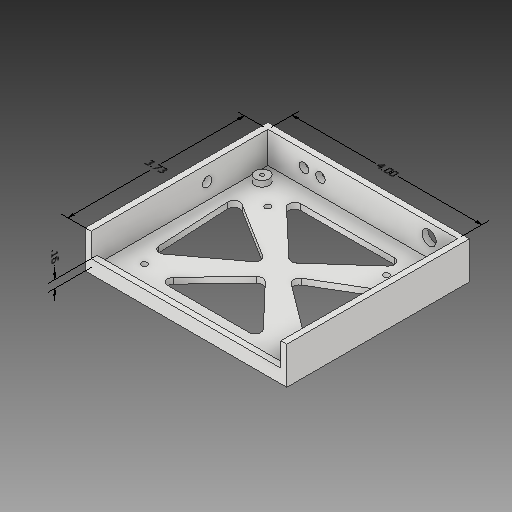
# Autodesk Inventor part: radiocase
Saved by Autodesk Inventor 2018 (Build 220112000, 112)
## iProperties
Created: 2018-03-21
Part Number: radiocase
Material: ABS Plastic
Document SubType Name: Modeling
Designer: Cole Tucker
Density: 1.06 g/cm^3
Appearance: Smooth - White
Mass: 40.9527 g
Surface Area: 278.233 cm^2
Volume: 38.6346 cm^3
Author: Cole Tucker
Autodesk Inventor part; units mm, degrees
ref_plane "YZ Plane" through (0, 0, 0) normal (1, 0, 0) x (0, 1, 0)
ref_plane "XZ Plane" through (0, 0, 0) normal (0, 1, 0) x (-1, 0, 0)
ref_plane "XY Plane" through (0, 0, 0) normal (0, 0, 1) x (1, 0, 0)
sketch "Sketch1" plane through (0, 0, 0) normal (0, 1, 0) x (-1, 0, 0)
  line L0 (0, 0) -> (3.175, 0)
  line L1 (3.175, 0) -> (3.175, -3.175)
  line L2 (3.175, -3.175) -> (0, -3.175)
  line L3 (0, -3.175) -> (0, 0)
  line L4 (3.175, -3.175) -> (104.775, -3.175)
  line L5 (104.775, -3.175) -> (104.775, -94.615)
  line L6 (104.775, -94.615) -> (3.175, -94.615)
  line L7 (3.175, -94.615) -> (3.175, -3.175)
  line L8 (104.775, -94.615) -> (107.95, -94.615)
  line L9 (107.95, -94.615) -> (107.95, -97.79)
  line L10 (107.95, -97.79) -> (104.775, -97.79)
  line L11 (104.775, -97.79) -> (104.775, -94.615)
  line L12 (107.95, -97.79) -> (0, -97.79)
  line L13 (0, -97.79) -> (0, 0)
  line L14 (0, 0) -> (107.95, 0)
  line L15 (107.95, 0) -> (107.95, -97.79)
  dimension "d0" = 3.175
  dimension "d1" = 3.175
  dimension "d2" = 101.6
  dimension "d3" = 91.44
  dimension "d4" = 3.175
  dimension "d5" = 3.175
  constraints: 32 end point, 8 parallel, 4 horizontal, 4 perpendicular
  measures "d0" distance of L1.end L2.end
  measures "d1" distance of L0.end L1.end
  measures "d2" distance of L5.end L6.end
  measures "d3" distance of L4.end L5.end
  measures "d4" distance of L9.end L10.end
  measures "d5" distance of L8.end L9.end
extrude "Extrusion1" add sketch "Sketch1" along normal blind 20 contours L0 L1 L2 L3 | L14 L15 L8 L5 L4 L1 | L2 L7 L6 L11 L12 L13 | L9 L10 L11 L8
sketch "Sketch6" plane through (0, 0, 0) normal (0, -1, 0) x (1, 0, 0)
  line L0 (-104.775, -3.175) -> (-3.175, -3.175) projected
  line L1 (-3.175, -3.175) -> (-3.175, -94.615) projected
  line L2 (-3.175, -94.615) -> (-104.775, -94.615) projected
  line L3 (-104.775, -94.615) -> (-104.775, -3.175) projected
  line L4 (0, 0) -> (0, -97.79) projected
  line L5 (-107.95, 0) -> (0, 0) projected
  line L6 (-107.95, -97.79) -> (-107.95, 0) projected
  line L7 (0, -97.79) -> (-107.95, -97.79) projected
extrude "Extrusion5" add sketch "Sketch6" against normal blind 3.175 contours L0 L1 L2 L3
sketch "Sketch7" plane through (0, 20, 0) normal (0, 1, 0) x (1, 0, 0)
  line L0 (-104.775, 3.175) -> (-3.175, 3.175)
  line L1 (-3.175, 3.175) -> (-3.175, 0)
  line L2 (-3.175, 0) -> (-104.775, 0)
  line L3 (-104.775, 0) -> (-104.775, 3.175)
  point P0 (0, 0)
  constraints: 8 end point, 2 parallel, 1 horizontal, 1 perpendicular
extrude "Extrusion6" cut sketch "Sketch7" against normal blind 12.7
sketch "Sketch9" plane through (0, 3.175, 0) normal (0, 1, 0) x (1, 0, 0)
  line L0 (-104.775, 94.615) -> (-3.175, 94.615) construction
  line L1 (-104.775, 94.615) -> (-101.473, 94.615) construction
  line L2 (-101.473, 94.615) -> (-101.473, 89.535) construction
  line L3 (-101.473, 89.535) -> (-104.775, 89.535) construction
  line L4 (-104.775, 89.535) -> (-104.775, 94.615) construction
  line L5 (-3.175, 94.615) -> (-3.175, 3.175) construction
  line L6 (-101.473, 89.535) -> (-3.175, 89.535) construction
  line L7 (-3.175, 89.535) -> (-3.175, 3.175) construction
  line L8 (-3.175, 3.175) -> (-101.473, 3.175) construction
  line L9 (-101.473, 3.175) -> (-101.473, 89.535) construction
  line L10 (-101.473, 89.535) -> (-98.933, 89.535) construction
  line L11 (-98.933, 89.535) -> (-98.933, 85.725) construction
  line L12 (-98.933, 85.725) -> (-101.473, 85.725) construction
  line L13 (-101.473, 85.725) -> (-101.473, 89.535) construction
  line L14 (-3.175, 89.535) -> (-6.985, 89.535) construction
  line L15 (-6.985, 89.535) -> (-6.985, 85.725) construction
  line L16 (-6.985, 85.725) -> (-3.175, 85.725) construction
  line L17 (-3.175, 85.725) -> (-3.175, 89.535) construction
  circle A0 centre (-98.933, 85.725) radius 3.81
  circle A1 centre (-6.985, 85.725) radius 3.81
  point P0 (0, 0)
  dimension "d53" = 3.302
  dimension "d54" = 5.08
  dimension "d55" = 2.54
  dimension "d56" = 3.81
  dimension "d57" = 3.81
  dimension "d58" = 3.81
  constraints: 32 end point, 8 parallel, 4 horizontal, 4 perpendicular, 2 coincident, 2 vertical alignment, 4 other
  measures "d53" distance of L2.end L3.end
  measures "d54" distance of L1.end L2.end
  measures "d55" distance of L11.end L12.end
  measures "d56" distance of L10.end L11.end
  measures "d57" distance of L16.end L15.end
  measures "d58" distance of L15.end L14.end
extrude "Extrusion9" add sketch "Sketch9" along normal blind 3.048
sketch "Sketch11" plane through (-104.775, 20, 0) normal (1, 0, 0) x (0, 0, -1)
  line L0 (89.535, -13.777) -> (81.915, -13.777) projected
  line L1 (85.725, -13.777) -> (62.103, -13.777)
  line L2 (62.103, -13.777) -> (62.103, -8.189)
  point P0 (0, -20)
  dimension "d103" = 5.588
  constraints: 4 end point, 1 horizontal, 1 midpoint
  measures "d103" distance of L1.end L2.end
hole "Hole3" at (-104.775, 11.811, -62.103) direction (-1, 0, 0) diameter 5.08 depth 4.064 tip angle 118
sketch "Sketch12" plane through (-98.933, 6.223, -85.725) normal (0, 1, 0) x (1, 0, 0)
  circle A0 centre (0, 0) radius 3.81 projected
  circle A1 centre (91.948, 0) radius 3.81 projected
  point P0 (98.933, -85.725)
  point P1 (95.758, 0)
  constraints: 2 coincident, 1 horizontal alignment
hole "Hole4" at (-98.933, 6.223, -85.725) at (-6.985, 6.223, -85.725) direction (0, -1, 0) diameter 2.032 depth 4.064 tip angle 118
sketch "Sketch13" plane through (-104.775, 20, -94.615) normal (0, 0, 1) x (1, 0, 0)
  line L0 (9.652, -13.777) -> (2.032, -13.777) projected
  line L1 (5.842, -13.777) -> (19.304, -13.777)
  line L2 (19.304, -13.777) -> (19.304, -8.189)
  line L3 (19.304, -8.189) -> (28.194, -8.189)
  point P0 (104.775, -20)
  dimension "d84" = 13.462
  dimension "d85" = 5.588
  dimension "d86" = 8.89
  constraints: 6 end point, 2 coincident, 2 perpendicular, 1 collinear, 1 midpoint
  measures "d84" distance of L1.start L1.end
  measures "d85" distance of L1.end L2.end
  measures "d86" distance of L2.end L3.end
hole "Hole5" at (-85.471, 11.811, -94.615) at (-76.581, 11.811, -94.615) direction (0, 0, -1) diameter 5.08 depth 4.064 tip angle 118
sketch "Sketch14" plane through (-104.775, 20, -94.615) normal (0, 0, 1) x (1, 0, 0)
  line L0 (0, -12.7) -> (101.6, -12.7) projected
  line L1 (101.6, -12.7) -> (101.6, -7.112)
  line L2 (101.6, -16.825) -> (101.6, 0) projected
  line L3 (101.6, -7.112) -> (86.36, -7.112)
  point P0 (104.775, -20)
  dimension "d94" = 5.588
  dimension "d95" = 15.24
  constraints: 4 end point, 1 coincident, 1 perpendicular, 1 point on line
  measures "d94" distance of L0.end L1.end
  measures "d95" distance of L1.end L3.end
hole "Hole6" at (-18.415, 12.888, -94.615) direction (0, 0, -1) diameter 7.62 depth 4.064 tip angle 118
sketch "Sketch15" plane through (0, 3.175, 0) normal (0, 1, 0) x (1, 0, 0)
  circle A0 centre (-98.933, 85.725) radius 1.016 projected
  line L0 (-98.933, 85.725) -> (-86.233, 85.725)
  circle A1 centre (-6.985, 85.725) radius 1.016 projected
  line L1 (-6.985, 85.725) -> (-19.685, 85.725)
  line L2 (-6.985, 85.725) -> (-6.985, 73.025)
  circle A2 centre (-98.933, 85.725) radius 3.81 projected
  line L3 (-98.933, 85.725) -> (-98.933, 73.025)
  line L4 (-104.775, 3.175) -> (-95.7947, 12.1553)
  line L5 (-104.775, 3.175) -> (-92.075, 3.175) construction
  line L6 (-3.175, 85.725) -> (-3.175, 3.175) projected
  line L7 (-3.175, 3.175) -> (-12.1553, 12.1553)
  line L8 (-3.175, 3.175) -> (9.525, 3.175) construction
  line L9 (-98.933, 73.025) -> (-95.7947, 12.1553)
  line L10 (-104.775, 0) -> (-104.775, 94.615) projected
  line L11 (-95.7947, 12.1553) -> (-12.1553, 12.1553)
  line L12 (-12.1553, 12.1553) -> (-6.985, 73.025)
  line L13 (-6.985, 73.025) -> (-19.685, 85.725)
  line L14 (-19.685, 85.725) -> (-86.233, 85.725)
  line L15 (-86.233, 85.725) -> (-98.933, 73.025)
  line L16 (-104.775, 94.615) -> (-3.175, 94.615) construction
  line L17 (-53.975, 94.615) -> (-53.975, 3.175) construction
  line L18 (-104.775, 3.175) -> (-3.175, 3.175) construction
  line L19 (-53.975, 48.895) -> (-60.325, 48.895) construction
  line L20 (-60.325, 48.895) -> (-60.325, 55.245) construction
  line L21 (-60.325, 55.245) -> (-53.975, 55.245) construction
  line L22 (-53.975, 55.245) -> (-53.975, 48.895) construction
  line L23 (-53.975, 48.895) -> (-47.625, 48.895) construction
  line L24 (-47.625, 48.895) -> (-47.625, 42.545) construction
  line L25 (-47.625, 42.545) -> (-53.975, 42.545) construction
  line L26 (-53.975, 42.545) -> (-53.975, 48.895) construction
  line L27 (-86.233, 85.725) -> (-53.975, 55.245)
  line L28 (-53.975, 55.245) -> (-19.685, 85.725)
  line L29 (-6.985, 73.025) -> (-47.625, 48.895)
  line L30 (-98.933, 73.025) -> (-60.325, 48.895)
  line L31 (-3.175, 3.175) -> (-3.175, 15.875) construction
  line L32 (-3.175, 3.175) -> (-15.875, 3.175) construction
  line L33 (-11.3251, 21.9293) -> (-47.625, 48.895)
  line L34 (-24.9577, 12.1553) -> (-53.975, 42.545)
  line L35 (-104.775, 3.175) -> (-92.075, 3.175) construction
  line L36 (-104.775, 3.175) -> (-104.775, 15.875) construction
  line L37 (-96.3107, 22.1628) -> (-60.325, 48.895)
  line L38 (-53.975, 42.545) -> (-83.3844, 12.1553)
  point P0 (0, 0)
  dimension "d104" = 12.7
  dimension "d105" = 12.7
  dimension "d106" = 12.7
  dimension "d107" = 12.7
  dimension "d108" = 12.7
  dimension "d109" = 45
  dimension "d110" = 12.7
  dimension "d111" = 135
  dimension "d112" = 6.35
  dimension "d113" = 6.35
  dimension "d114" = 6.35
  dimension "d115" = 6.35
  dimension "d116" = 12.7
  dimension "d117" = 12.7
  dimension "d118" = 12.7
  dimension "d119" = 12.7
  constraints: 70 end point, 7 point on line, 6 horizontal, 5 parallel, 3 midpoint, 3 perpendicular, 2 equal length, 2 vertical, 1 collinear
  measures "d104" distance of L0.start L0.end
  measures "d105" distance of L1.start L1.end
  measures "d106" distance of L1.start L2.end
  measures "d107" distance of L3.start L3.end
  measures "d108" distance of L4.start L4.end
  measures "d109" angle of L5 L4
  measures "d110" distance of L6.end L7.end
  measures "d111" angle of L8 L7
  measures "d112" distance of L20.end L21.end
  measures "d113" distance of L19.end L20.end
  measures "d114" distance of L24.end L25.end
  measures "d115" distance of L23.end L24.end
  measures "d116" distance of L6.end L31.end
  measures "d117" distance of L6.end L32.end
  measures "d118" distance of L4.start L5.end
  measures "d119" distance of L4.start L36.end
extrude "Extrusion10" cut sketch "Sketch15" against normal blind 25.4 contours L14 L28 L27 | L30 L37 L9 | L12 L33 L29 | L38 L34 L11
fillet "Fillet1" radius 3.175 12 edges at (-96.3107, 1.5875, -22.1628) (-60.325, 1.5875, -48.895) (-53.975, 1.5875, -55.245) (-53.975, 1.5875, -42.545) (-47.625, 1.5875, -48.895) (-83.3844, 1.5875, -12.1553) (-24.9577, 1.5875, -12.1553) (-86.233, 1.5875, -85.725) (-98.933, 1.5875, -73.025) (-19.685, 1.5875, -85.725) (-6.985, 1.5875, -73.025) (-11.3251, 1.5875, -21.9293)
sketch "Sketch16" plane through (0, 3.175, 0) normal (0, 1, 0) x (1, 0, 0)
  line L0 (-104.775, 3.175) -> (-104.775, 94.615) construction
  line L1 (-104.775, 94.615) -> (-85.725, 94.615) construction
  line L2 (-85.725, 94.615) -> (-85.725, 75.565) construction
  line L3 (-85.725, 75.565) -> (-104.775, 75.565) construction
  line L4 (-104.775, 75.565) -> (-104.775, 94.615) construction
  line L5 (-3.175, 94.615) -> (-22.225, 94.615) construction
  line L6 (-22.225, 94.615) -> (-22.225, 75.565) construction
  line L7 (-22.225, 75.565) -> (-3.175, 75.565) construction
  line L8 (-3.175, 75.565) -> (-3.175, 94.615) construction
  line L9 (-3.175, 3.175) -> (-104.775, 3.175) construction
  line L10 (-104.775, 3.175) -> (-92.075, 3.175) construction
  line L11 (-92.075, 3.175) -> (-92.075, 15.875) construction
  line L12 (-92.075, 15.875) -> (-104.775, 15.875) construction
  line L13 (-104.775, 15.875) -> (-104.775, 3.175) construction
  line L14 (-3.175, 3.175) -> (-15.875, 3.175) construction
  line L15 (-15.875, 3.175) -> (-15.875, 15.875) construction
  line L16 (-15.875, 15.875) -> (-3.175, 15.875) construction
  line L17 (-3.175, 15.875) -> (-3.175, 3.175) construction
  point P0 (0, 0)
  dimension "d123" = 19.05
  dimension "d124" = 19.05
  dimension "d125" = 19.05
  dimension "d126" = 19.05
  dimension "d127" = 12.7
  dimension "d128" = 12.7
  dimension "d129" = 12.7
  dimension "d130" = 12.7
  constraints: 32 end point, 8 parallel, 4 coincident, 4 horizontal, 4 perpendicular
  measures "d123" distance of L2.end L3.end
  measures "d124" distance of L1.end L2.end
  measures "d125" distance of L7.end L6.end
  measures "d126" distance of L5.end L6.end
  measures "d127" distance of L12.end L11.end
  measures "d128" distance of L11.end L10.end
  measures "d129" distance of L15.end L16.end
  measures "d130" distance of L14.end L15.end
hole "Hole7" at (-3.175, 3.175, -94.615) at (-85.725, 3.175, -75.565) at (-22.225, 3.175, -75.565) at (-15.875, 3.175, -15.875) at (-92.075, 3.175, -15.875) direction (0, -1, 0) diameter 3.175 depth 25.4 tip angle 118
body "Solid1"
